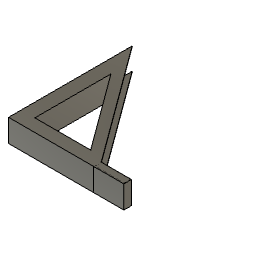
Pill Holder complete (Autodesk Fusion 360 design; units mm, degrees)
Autodesk Fusion 360 part; units mm, degrees
sketch "Sketch1" plane through (0, 0, 0) normal (0, 0, 1) x (1, 0, 0)
  line L0 (30, -40.9) -> (-30, -40.9)
  line L1 (-30, -40.9) -> (-30, 40.9)
  line L2 (-30, 40.9) -> (30, 40.9)
  line L3 (30, 40.9) -> (30, -40.9)
  line L4 (30, -40.9) -> (-30, 40.9) construction
  line L5 (-30, -40.9) -> (30, 40.9) construction
  line L6 (-30, 40.9) -> (30, -40.9)
  dimension "d1" = 60
  dimension "d2" = 81.8
  constraint horizontal L0
  constraint perpendicular L0 L1
  constraint parallel L0 L2
  constraint parallel L1 L3
  constraint coincident L4 origin
  constraint coincident L5 origin
  measures "d1" distance of L1.end L2.end
  measures "d2" distance of L0.end L1.end
extrude "Extrude1" add sketch "Sketch1" along normal blind 15 contours L0 L1 L6 makes body 1
sketch "Sketch2" plane through (0, 0, 0) normal (0.806342, 0.591449, 0) x (-0.591449, 0.806342, 0)
  line L0 (-50.7229, 0) -> (50.7229, 0)
  line L1 (50.7229, 0) -> (50.7229, 15)
  line L2 (50.7229, 15) -> (-50.7229, 15)
  line L3 (-50.7229, 15) -> (-50.7229, 0)
  line L4 (51, 14.5) -> (-51, 14.5)
  line L5 (-51, 14.5) -> (-51, 0.5)
  line L6 (-51, 0.5) -> (51, 0.5)
  line L7 (51, 0.5) -> (51, 14.5)
  line L8 (51, 14.5) -> (-51, 0.5) construction
  line L9 (-51, 14.5) -> (51, 0.5) construction
  point P0 (0, 7.5)
  dimension "d5" = 102
  dimension "d6" = 14
  constraint horizontal L4
  constraint perpendicular L4 L5
  constraint parallel L4 L6
  constraint parallel L5 L7
  constraint coincident L8 P0
  constraint coincident L9 P0
  measures "d5" distance of L5.end L6.end
  measures "d6" distance of L4.end L5.end
extrude "Extrude2" cut sketch "Sketch2" against normal blind 3 contours L1 L3 L4 L6 bodies 1
sketch "Sketch3" plane through (0, 0, 15) normal (0, 0, 1) x (-1, 0, 0)
  line L0 (30, -40.9) -> (30, 40.9)
  line L1 (30, 40.9) -> (-30, 40.9)
  line L2 (-30, 40.9) -> (30, -40.9)
  line L3 (21, 32.5) -> (-21, 32.5)
  line L4 (-21, 32.5) -> (-21, -32.5)
  line L5 (-21, -32.5) -> (21, -32.5)
  line L6 (21, -32.5) -> (21, 32.5)
  line L7 (21, 32.5) -> (-21, -32.5) construction
  line L8 (-21, 32.5) -> (21, -32.5) construction
  line L9 (21, -17.8629) -> (-15.941, 32.5)
  dimension "d9" = 42
  dimension "d10" = 65
  constraint horizontal L3
  constraint perpendicular L3 L4
  constraint parallel L3 L5
  constraint parallel L4 L6
  constraint coincident L7 origin
  constraint coincident L8 origin
  constraint coincident L6 L9.start
  constraint coincident L3 L9.end
  constraint parallel L2 L9
  measures "d9" distance of L4.end L5.end
  measures "d10" distance of L3.end L4.end
extrude "Extrude3" cut sketch "Sketch3" against normal blind 25 contours L3 L6 L9 bodies 1
sketch "Sketch4" plane through (0, -40.9, 0) normal (0, -1, 0) x (1, 0, 0)
  line L0 (26.2795, 14.5) -> (30, 14.5)
  line L1 (30, 14.5) -> (30, 15)
  line L2 (30, 15) -> (-30, 15)
  line L3 (-30, 15) -> (-30, 0)
  line L4 (-30, 0) -> (30, 0)
  line L5 (30, 0) -> (30, 0.5)
  line L6 (30, 0.5) -> (26.2795, 0.5)
  line L7 (26.2795, 0.5) -> (26.2795, 14.5)
  line L8 (26.2795, 14.5) -> (46.2795, 14.5)
  line L9 (46.2795, 14.5) -> (46.2795, 0.5)
  line L10 (46.2795, 0.5) -> (26.2795, 0.5)
  line L11 (26.2795, 0.5) -> (26.2795, 14.5)
  dimension "d13" = 20
  dimension "d14" = 14
  constraint horizontal L8
  constraint vertical L9
  constraint horizontal L10
  constraint vertical L11
  constraint coincident L0.start L7.end
  measures "d13" distance of L0.start L8.end
  measures "d14" distance of L0.start L6.end
extrude "Extrude4" add sketch "Sketch4" against normal blind 10 separate body contours L0 L6 L7 L8 L9 L10 L11 makes body 2
sketch "Sketch5" plane through (0, -30.9, 0) normal (0, 1, 0) x (-1, 0, 0)
  line L0 (-46.2795, 0.5) -> (-26.2795, 0.5)
  line L1 (-26.2795, 0.5) -> (-26.2795, 14.5)
  line L2 (-26.2795, 14.5) -> (-46.2795, 14.5)
  line L3 (-46.2795, 14.5) -> (-46.2795, 0.5)
  line L4 (-45.5988, 14.4934) -> (-24.9517, 14.4934)
  line L5 (-24.9517, 14.4934) -> (-24.9517, 0.5954)
  line L6 (-24.9517, 0.5954) -> (-45.5988, 0.5954)
  line L7 (-45.5988, 0.5954) -> (-45.5988, 14.4934)
  constraint horizontal L4
  constraint vertical L5
  constraint horizontal L6
  constraint vertical L7
extrude "Extrude5" cut sketch "Sketch5" against normal blind 9 contours L1 L4 L6 L7 | L1 L4 L5 L6 bodies 2
move_face "OffsetFaces1" offset 0.5 1 faces at (32.9462, -37.5667, 14.5) on bodies 2
sketch "Sketch6" plane through (0, 0, 15) normal (0, 0, 1) x (-1, 0, 0)
  line L0 (-26.2795, 40.9) -> (-46.2795, 40.9)
  line L1 (-46.2795, 40.9) -> (-46.2795, 30.9)
  line L2 (-46.2795, 30.9) -> (-26.2795, 30.9)
  line L3 (-26.2795, 30.9) -> (-26.2795, 40.9)
  line L4 (-26.2795, 35.9) -> (-46.2795, 35.9)
  constraint midpoint L3 L4.start
  constraint midpoint L1 L4.end
extrude "Extrude6" cut sketch "Sketch6" against normal blind 22 contours L1 L2 L3 L4 bodies 1 2
move_face "OffsetFaces2" offset 0.5 1 faces at (39.6128, -39.2333, 0.5) on bodies 2
combine "Combine1" operation add target body 2 tool bodies 1
equation "d20 = -2 mm - 20 mm"
